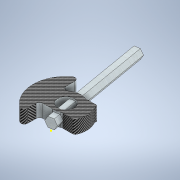
# Autodesk Inventor part: Hacha_01
Saved by Autodesk Inventor 2022.2 (Build 262287010, 287A)
## iProperties
Created: 2022-03-11
Part Number: Hacha_01
Material: Generic
Document SubType Name: Modeling
Designer: Santiago Larraín
Density: 1 g/cm^3
Appearance: Default
Author: Santiago Larraín
Autodesk Inventor part; units mm, degrees
ref_plane "YZ Plane" through (0, 0, 0) normal (1, 0, 0) x (0, 1, 0)
sketch "Sketch1" plane through (0, 0, 0) normal (0, 1, 0) x (-1, 0, 0)
  line L0 (-27.111, 15.2395) -> (22.2425, -12.5029) construction
  line L1 (22.6574, 17.4943) -> (-27.0498, -20.8857) construction
  line L2 (0, 0) -> (50, 0)
  arc A0 (22.2425, -44.7803) -> (22.6574, 44.5718) centre (0, 0) ccw
  arc A1 (2.535, 17.4943) -> (-8.9573, 15.2395) centre (0, 0) ccw
  arc A2 (-27.111, 16.0519) -> (-27.0498, -16.1549) centre (0, 0) ccw
  arc A3 (-9.006, -20.8857) -> (19, -12.5029) centre (0, 0) ccw
  line L3 (22.6574, 17.4943) -> (22.6574, 44.5718)
  line L4 (22.2425, -44.7803) -> (22.2425, -12.5029)
  line L5 (-27.111, 15.2395) -> (-8.9573, 15.2395)
  line L6 (2.535, 17.4943) -> (22.6574, 17.4943)
  line L7 (22.2425, -12.5029) -> (19, -12.5029)
  line L8 (-9.006, -20.8857) -> (-27.0498, -20.8857)
  line L9 (-27.0498, -20.8857) -> (-27.0498, -16.1549)
  line L10 (-27.111, 16.0519) -> (-27.111, 15.2395)
  dimension "d1" = 30
  dimension "d2" = 50
  dimension "d3" = 50
  constraints: 22 end point, 9 point on circle, 8 parallel, 4 centre point, 4 perpendicular, 3 horizontal, 2 point on line, 1 coincident
  measures "d1" distance of L1.start L0.end
  measures "d2" distance of L0.end L1.end
  measures "d3" distance of L2.start L2.end
extrude "Extrusion1" add sketch "Sketch1" along normal blind 20
sketch "Sketch2" plane through (0, 20, 0) normal (0, 1, 0) x (1, 0, 0)
  circle A0 centre (0, 0) radius 12.5
  dimension "d6" = 25
  constraints: 1 centre point, 1 coincident
  measures "d6" diameter of A0
extrude "Extrusion2" cut sketch "Sketch2" against normal through all
fillet "Fillet1" radius 2 2 edges at (27.111, 10, 15.2395) (27.0498, 10, -20.8857)
fillet "Fillet2" radius 5 10 edges at (-22.2425, 10, -12.5029) (-22.6574, 10, 17.4943) (-22.2425, 10, -44.7803) (-19, 10, -12.5029) (-22.6574, 10, 44.5718) (9.006, 10, -20.8857) (-2.535, 10, 17.4943) (8.9573, 10, 15.2395) (27.111, 10, 16.0519) (27.0498, 10, -16.1549)
ref_plane "Work Plane1" through (2.9983, 0, 17.4209) normal (0.1696154, 0, 0.9855103) x (0, 1, 0)
sketch "Sketch3" plane through (0, 0, 0) normal (0, -1, 0) x (1, 0, 0)
  point P0 (0, 0)
ref_plane "Work Plane2" through (2.9983, 0, 17.4209) normal (0.1696154, 0, 0.9855103) x (0, 1, 0)
sketch "Sketch4" plane through (0, 10, 0) normal (0, 1, 0) x (1, 0, 0)
  point P0 (0, 0)
sketch "Sketch5" plane through (2.9983, 0, 17.4209) normal (0.1696154, 0, 0.9855103) x (0, 1, 0)
  line L0 (10, 12.5) -> (10, -12.5) projected
  line L1 (10, -8.3729) -> (2.7489, -4.1864)
  line L2 (2.7489, -4.1864) -> (2.7489, 4.1864)
  line L3 (2.7489, 4.1864) -> (10, 8.3729)
  line L4 (10, 8.3729) -> (17.2511, 4.1864)
  line L5 (17.2511, 4.1864) -> (17.2511, -4.1864)
  line L6 (17.2511, -4.1864) -> (10, -8.3729)
  point P0 (0, 0)
  point P1 (10, 0)
  constraints: 12 end point, 1 midpoint, 1 point on line, 13 other
extrude "Extrusion3" add sketch "Sketch5" along normal blind 10 and the other way blind 150
sketch "Sketch6" plane through (4.6944, 0, 27.276) normal (0.1696154, 0, 0.9855103) x (0.9855103, 0, -0.1696154)
  point P0 (0, 0)
body "Solid1"
